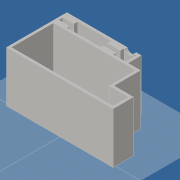
# Autodesk Inventor part: Erweiterung
Saved by Autodesk Inventor 2016 SP2 (Build 200236200, 236)
## iProperties
Created: 2018-07-08
Part Number: Erweiterung
Material: Generisch
Document SubType Name: Modeling
Designer: User
Density: 1 g/cm^3
Appearance: Vorgabe
Author: User
Autodesk Inventor part; units mm, degrees
ref_plane "YZ Plane" through (0, 0, 0) normal (1, 0, 0) x (0, 1, 0)
ref_plane "XZ Plane" through (0, 0, 0) normal (0, 1, 0) x (-1, 0, 0)
ref_plane "XY Plane" through (0, 0, 0) normal (0, 0, 1) x (1, 0, 0)
sketch "Skizze1" plane through (0, 0, 0) normal (0, 0, 1) x (1, 0, 0)
  line L0 (-65, 0) -> (65, 0)
  line L1 (65, 0) -> (65, 20)
  line L2 (65, 20) -> (40, 20)
  line L3 (40, 20) -> (40, 54)
  line L4 (-65, 41) -> (-65, 0)
  line L5 (-65, 41) -> (-65, 41)
  line L6 (-65, 54) -> (-65, 54)
  line L7 (-65, 54) -> (-65, 41)
  line L8 (24, 71) -> (24, 54)
  line L9 (24, 54) -> (40, 54)
  line L10 (-65, 54) -> (24, 54)
  line L11 (24, 54) -> (24, 57)
  line L12 (24, 57) -> (-65, 57)
  line L13 (-65, 57) -> (-65, 54)
  line L14 (24, 71) -> (-65, 71)
  line L15 (-65, 71) -> (-65, 54)
  line L16 (43, 23) -> (68, 23)
  line L17 (68, 23) -> (68, -3)
  line L18 (68, -3) -> (-68, -3)
  line L19 (-68, -3) -> (-68, 44)
  line L20 (-68, 44) -> (-68, 44)
  line L21 (-68, 44) -> (-68, 57)
  line L22 (-68, 57) -> (-68, 57)
  line L23 (-68, 57) -> (-68, 74)
  line L24 (-68, 74) -> (27, 74)
  line L25 (27, 74) -> (27, 57)
  line L26 (27, 57) -> (43, 57)
  line L27 (43, 57) -> (43, 23)
  line L28 (-65, 71) -> (-51, 71)
  line L29 (-51, 71) -> (-51, 66)
  line L30 (-51, 66) -> (-65, 66)
  line L31 (-65, 66) -> (-65, 71)
  line L32 (8, 71) -> (-8, 71)
  line L33 (-8, 71) -> (-8, 66)
  line L34 (-8, 66) -> (8, 66)
  line L35 (8, 66) -> (8, 71)
  line L36 (-65, 71) -> (-55, 71)
  line L37 (-55, 71) -> (-55, 66)
  line L38 (-55, 66) -> (-65, 66)
  line L39 (-65, 66) -> (-65, 71)
  line L40 (1, 71) -> (-4, 71)
  line L41 (-4, 71) -> (-4, 66)
  line L42 (-4, 66) -> (1, 66)
  line L43 (1, 66) -> (1, 71)
  line L44 (8, 71) -> (1, 71)
  line L45 (1, 71) -> (1, 66)
  line L46 (1, 66) -> (8, 66)
  line L47 (8, 66) -> (8, 71)
  line L48 (-4, 71) -> (-8, 71)
  line L49 (-8, 71) -> (-8, 66)
  line L50 (-8, 66) -> (-4, 66)
  line L51 (-4, 66) -> (-4, 71)
  line L52 (8, 57) -> (-8, 57)
  line L53 (-8, 57) -> (-8, 60.5)
  line L54 (-8, 60.5) -> (8, 60.5)
  line L55 (8, 60.5) -> (8, 57)
  line L56 (1, 60.5) -> (-4, 60.5)
  line L57 (-4, 60.5) -> (-4, 57)
  line L58 (-4, 57) -> (1, 57)
  line L59 (1, 57) -> (1, 60.5)
  line L60 (-65, 57) -> (-51, 57)
  line L61 (-51, 57) -> (-51, 60.5)
  line L62 (-51, 60.5) -> (-65, 60.5)
  line L63 (-65, 60.5) -> (-65, 57)
  line L64 (-55, 60.5) -> (-65, 60.5)
  line L65 (-65, 60.5) -> (-65, 57)
  line L66 (-65, 57) -> (-55, 57)
  line L67 (-55, 57) -> (-55, 60.5)
  line L68 (-65, 57) -> (24, 57)
  line L69 (24, 57) -> (24, 54)
  line L70 (24, 54) -> (-65, 54)
  line L71 (-65, 54) -> (-65, 57)
  point P0 (0, 0)
  point P1 (0, 0)
  point P2 (0, 0)
  point P3 (0, 0)
  dimension "d0" = 130
  dimension "d1" = 25
  dimension "d2" = 20
  dimension "d3" = 41
  dimension "d4" = 54
  dimension "d16" = 0
  dimension "d17" = 89
  dimension "d18" = 71
  dimension "d19" = 3
  dimension "d21" = 16
  dimension "d22" = 14
  dimension "d23" = 5
  dimension "d24" = 43
  dimension "d25" = 10
  dimension "d26" = 51
  dimension "d27" = 5
  dimension "d28" = 5.5
  dimension "d31" = 3
  dimension "d41" = 0
  constraints: 145 end point, 24 parallel, 22 perpendicular, 16 horizontal, 10 point on line, 9 collinear, 3 coincident, 1 midpoint, 1 vertical, 11 other
  measures "d0" distance between parallel lines of L1 L4
  measures "d1" distance between parallel lines of L1 L3
  measures "d2" distance between parallel lines of L0 L2
  measures "d3" distance between parallel lines of L0 L5
  measures "d4" distance between parallel lines of L0 L6
  measures "d16" distance between parallel lines of L7 L4
  measures "d17" distance of L8.start L14.end
  measures "d18" distance between parallel lines of L0 L14
  measures "d19" distance between parallel lines of L2 L16
  measures "d21" distance of L33.end L34.end
  measures "d22" distance of L29.end L30.end
  measures "d23" distance of L34.end L32.start
  measures "d24" distance between parallel lines of L29 L33
  measures "d25" distance between parallel lines of L15 L37
  measures "d26" distance between parallel lines of L37 L41
  measures "d27" distance between parallel lines of L41 L43
  measures "d28" distance between parallel lines of L54 L46
  measures "d31" distance between parallel lines of L10 L12
  measures "d41" distance between parallel lines of L23 L21
extrude "Extrusion1" add sketch "Skizze1" against normal blind 3 contours L4 L7 L10 L9 L3 L2 L1 L0 | L13 L12 L8 L10 | L15 L62 L67 L12 | L12 L55 L54 L53 L61 L62 L15 L30 L29 L14 L33 L34 L35 L8 | L67 L62 L61 L12 | L12 L59 L54 L55 | L15 L14 L37 L30 | L35 L34 L43 L14 | L12 L57 L54 L59 | L53 L54 L57 L12 | L37 L14 L29 L30 | L43 L34 L41 L14 | L41 L34 L33 L14 | L16 L17 L18 L19 L21 L23 L24 L25 L26 L27
extrude "Extrusion2" add sketch "Skizze1" along normal blind 62 contours L13 L12 L8 L10 | L15 L62 L67 L12 | L67 L62 L61 L12 | L12 L59 L54 L55 | L15 L14 L37 L30 | L35 L34 L43 L14 | L12 L57 L54 L59 | L53 L54 L57 L12 | L37 L14 L29 L30 | L43 L34 L41 L14 | L41 L34 L33 L14 | L16 L17 L18 L19 L21 L23 L24 L25 L26 L27
sketch "Skizze2" plane through (-68, 74, -3) normal (0, 1, 0) x (1, 0, 0)
  line L0 (95, -65) -> (95, 0) projected
  line L1 (95, -65) -> (0, -65) projected
  line L2 (92, -65) -> (76, -65) projected
  arc A0 (88.5, -65) -> (77, -65) centre (82.75, -66.7139) ccw
  line L3 (77, -65) -> (88.5, -65)
  point P0 (68, -3)
  dimension "d36" = 6
  dimension "d37" = 12.25
  dimension "d38" = 11.5
  constraints: 2 end point, 2 point on circle, 2 point on line, 1 centre point, 1 collinear
  measures "d36" radius of A0
  measures "d37" distance from line of L0 A0.centre
  measures "d38" distance of L3.end L3.start
extrude "Extrusion3" cut sketch "Skizze2" against normal up to surface (3 mm away)
